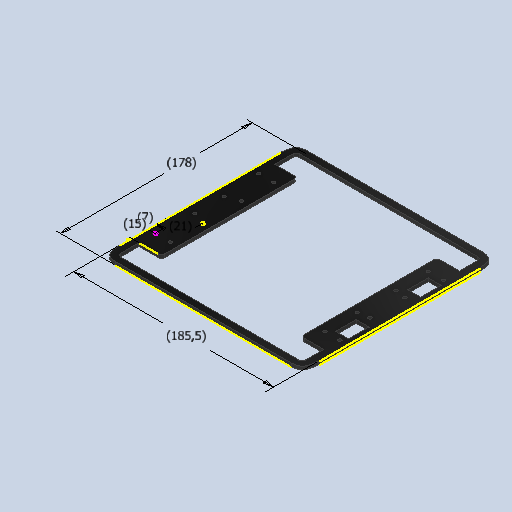
# Autodesk Inventor part: rama
Saved by Autodesk Inventor 2022 (Build 260153000, 153)
## iProperties
Created: 2022-07-21
Part Number: rama
Material: Серебро
Document SubType Name: Modeling
Designer: akapu
Density: 10.49 g/cm^3
Appearance: Серебро
Author: akapu
Autodesk Inventor part; units mm, degrees
ref_plane "YZ Plane" through (0, 0, 0) normal (1, 0, 0) x (0, 1, 0)
ref_plane "XZ Plane" through (0, 0, 0) normal (0, 1, 0) x (-1, 0, 0)
ref_plane "XY Plane" through (0, 0, 0) normal (0, 0, 1) x (1, 0, 0)
sketch "Эскиз1" plane through (0, 0, 0) normal (0, 1, 0) x (-1, 0, 0)
  line L0 (0, 0) -> (-92.765, 0)
  line L1 (-92.765, 0) -> (-92.765, -66)
  line L2 (-92.765, -66) -> (0, -66)
  line L3 (0, -66) -> (0, 0)
  line L4 (0, 0) -> (-43, 0)
  line L5 (-43, 0) -> (-43, 1)
  line L6 (-43, 1) -> (-6, 1)
  line L7 (-6, 1) -> (-6, 16)
  line L8 (-6, 16) -> (-80, 16)
  line L9 (-80, 16) -> (-80, 1)
  line L10 (-80, 1) -> (-43, 1)
  line L11 (0, 0) -> (0, 17)
  line L12 (0, 17) -> (-92.765, 17)
  line L13 (-92.765, 17) -> (-92.765, 0)
  line L14 (0, 17) -> (0, 23)
  line L15 (0, 23) -> (-92.765, 23)
  line L16 (-92.765, 23) -> (-92.765, 17)
  line L17 (-43, 16) -> (-43, 23)
  line L18 (0, 0) -> (-7, 0)
  line L19 (-7, 0) -> (-7, 17)
  line L20 (0, 0) -> (-8, 0)
  line L21 (-8, 0) -> (-8, -3)
  line L22 (-8, -3) -> (-92.765, -3)
  line L23 (-8, -3) -> (-8, -66)
  line L24 (-7, 17) -> (0, 23)
  line L25 (-3.5, 20) -> (-0.0714, 16)
  line L26 (-0.0714, 16) -> (-6.0714, 23)
  line L27 (0, 15.9167) -> (-3.5, 20)
  line L28 (-3.5, 20) -> (-6.0714, 23)
  spline S0 degree 3 poles (0, 8.5) (-1.6685, 20.9552) (-1.0245, 23.9091) (-21.5, 23) knots 0 0 0 0 1 1 1 1
  point P0 (-1.75, 17.9583)
  point P1 (-4.7857, 21.5)
  point P2 (-11.0558, 23)
  dimension "d68" = 43
  dimension "d71" = 1
  dimension "d72" = 37
  dimension "d74" = 74
  dimension "d75" = 17
  dimension "d76" = 6
  dimension "d77" = 7
  dimension "d78" = 8
  dimension "d79" = 3
  constraints: 58 end point, 15 point on line, 13 perpendicular, 6 midpoint, 3 parallel, 2 collinear, 2 horizontal, 4 other
  measures "d68" distance of L0.start L4.end
  measures "d71" distance of L4.end L5.end
  measures "d72" distance of L5.end L6.end
  measures "d74" distance of L7.end L8.end
  measures "d75" distance of L0.start L11.end
  measures "d76" distance of L11.end L14.end
  measures "d77" distance of L0.start L18.end
  measures "d78" distance of L0.start L20.end
  measures "d79" distance of L20.end L21.end
extrude "Выдавливание2" add sketch "Эскиз1" against normal blind 3 contours L3 L2 L23 L21 L0 | L0 L19 L6 L7 L8 L12 S0 L11 | L19 L8 L7 L6 | L12 L24 L25 S0 | L12 L17 L15 S0 L26 L24 | L25 L24 S0 | L12 L16 L15 L17 | L26 S0 L24
mirror "Зеркальное отражение1" about plane through (0, 0, -66) normal (0, 0, -1) of "Выдавливание2"
mirror "Зеркальное отражение2" about plane through (92.765, 0, -149) normal (1, 0, 0) of "Выдавливание2", "Зеркальное отражение1"
fillet "Сопряжение2" radius 3 4 edges at (7, -1.5, 17) (178.53, -1.5, 17) (178.53, -1.5, -149) (7, -1.5, -149)
sketch "Эскиз4" plane through (0, -3, 0) normal (0, -1, 0) x (1, 0, 0)
  line L0 (174.4742, -155) -> (11.0558, -155) projected
  line L1 (11.0558, 23) -> (174.4742, 23) projected
  line L2 (185.53, -140.5) -> (185.53, 8.5) projected
  line L3 (0, 8.5) -> (0, -140.5) projected
  point P0 (0, 0)
  dimension "d87" = 178
  measures "d87" distance between parallel lines of L0 L1
sketch "Эскиз5" plane through (0, 0, 0) normal (0, 1, 0) x (1, 0, 0)
  line L0 (8, 0) -> (8, 132) projected
  line L1 (8, 0) -> (8, 3)
  line L2 (8, 3) -> (177.53, 3)
  line L3 (177.53, 0) -> (177.53, 132) projected
  line L4 (8, 132.1275) -> (8, 129.1275)
  line L5 (8, 129.1275) -> (177.53, 129.1275)
  line L6 (8, 129.1275) -> (28, 129.1275)
  line L7 (28, 129.1275) -> (28, 3)
  line L8 (28, 3) -> (8, 3)
  line L9 (8, 3) -> (8, 129.1275)
  line L10 (177.53, 129.1275) -> (157.53, 129.1275)
  line L11 (157.53, 129.1275) -> (157.53, 3)
  line L12 (157.53, 3) -> (177.53, 3)
  line L13 (177.53, 3) -> (177.53, 129.1275)
  line L14 (28, 129.1275) -> (14, 129.1275)
  line L15 (14, 129.1275) -> (14, 3)
  line L16 (157.53, 129.1275) -> (171.53, 129.1275)
  line L17 (171.53, 129.1275) -> (171.53, 3)
  line L18 (164.53, 3) -> (164.53, 18)
  line L19 (164.53, 18) -> (178.53, 18)
  line L20 (164.53, 18) -> (164.53, 48)
  line L21 (164.53, 48) -> (178.53, 48)
  line L22 (185.53, 140.5) -> (185.53, -8.5) projected
  line L23 (178.53, 48) -> (178.53, 18)
  line L24 (164.53, 129.1275) -> (164.53, 114.1275)
  line L25 (164.53, 114.1275) -> (164.53, 84.1275)
  line L26 (164.53, 84.1275) -> (178.53, 84.1275)
  line L27 (178.53, 84.1275) -> (178.53, 114.1275)
  line L28 (178.53, 114.1275) -> (164.53, 114.1275)
  line L29 (21, 129.1275) -> (21, 114.1275)
  line L30 (21, 114.1275) -> (21, 84.1275)
  line L31 (21, 3) -> (21, 18)
  line L32 (21, 18) -> (21, 48)
  line L33 (21, 48) -> (7, 48)
  line L34 (21, 18) -> (7, 18)
  line L35 (7, 18) -> (7, 48)
  line L36 (21, 84.1275) -> (7, 84.1275)
  line L37 (7, 84.1275) -> (7, 114.1275)
  line L38 (7, 114.1275) -> (21, 114.1275)
  circle A0 centre (7, 114.1275) radius 1.5
  circle A1 centre (21, 114.1275) radius 1.5
  circle A2 centre (21, 84.1275) radius 1.5
  circle A3 centre (7, 18) radius 1.5
  circle A4 centre (21, 18) radius 1.5
  circle A5 centre (21, 48) radius 1.5
  circle A6 centre (164.53, 114.1275) radius 1.5
  circle A7 centre (178.53, 114.1275) radius 1.5
  circle A8 centre (178.53, 84.1275) radius 1.5
  circle A9 centre (164.53, 84.1275) radius 1.5
  circle A10 centre (164.53, 48) radius 1.5
  circle A11 centre (178.53, 48) radius 1.5
  circle A12 centre (178.53, 18) radius 1.5
  circle A13 centre (164.53, 18) radius 1.5
  arc A14 (10.584, 53.1837) -> (8.6151, 50.9779) centre (9.41, 52.25) ccw projected
  arc A15 (8.6151, 50.9779) -> (10.584, 53.1837) centre (9.41, 52.25) ccw projected
  arc A16 (10.584, 78.8163) -> (8.6151, 81.0221) centre (9.41, 79.75) ccw projected
  arc A17 (8.6151, 81.0221) -> (10.584, 78.8163) centre (9.41, 79.75) ccw projected
  arc A18 (8.6151, 81.0221) -> (10.584, 78.8163) centre (9.41, 79.75) ccw projected
  circle A19 centre (9.41, 52.25) radius 1.5
  circle A20 centre (9.41, 79.75) radius 1.5
  point P0 (0, 0)
  point P1 (177.53, 16.882)
  point P2 (177.53, 19.118)
  point P3 (177.53, 46.882)
  point P4 (177.53, 49.118)
  point P5 (177.53, 83.0095)
  point P6 (177.53, 85.2455)
  point P7 (177.53, 113.0095)
  point P8 (177.53, 115.2455)
  point P9 (8, 115.2455)
  point P10 (8, 113.0095)
  point P11 (8, 19.118)
  point P12 (8, 16.882)
  point P13 (8, 80.2618)
  point P14 (8, 79.2382)
  point P15 (8, 52.7618)
  point P16 (8, 51.7382)
  dimension "d90" = 3
  dimension "d91" = 3
  dimension "d92" = 20
  dimension "d93" = 20
  dimension "d94" = 14
  dimension "d95" = 14
  dimension "d96" = 15
  dimension "d97" = 14
  dimension "d98" = 30
  dimension "d99" = 15
  dimension "d100" = 30
  dimension "d101" = 15
  dimension "d102" = 30
  dimension "d103" = 15
  dimension "d104" = 30
  dimension "d105" = 14
  dimension "d106" = 14
  dimension "d107" = 14
  dimension "d108" = 3
  dimension "d109" = 3
  dimension "d110" = 3
  dimension "d112" = 3
  dimension "d113" = 3
  dimension "d114" = 3
  dimension "d116" = 3
  dimension "d117" = 3
  dimension "d118" = 3
  dimension "d119" = 3
  dimension "d120" = 3
  dimension "d121" = 3
  dimension "d122" = 3
  dimension "d123" = 3
  constraints: 72 end point, 17 point on line, 16 centre point, 16 coincident, 16 perpendicular, 6 parallel, 3 horizontal, 2 concentric, 2 midpoint, 1 vertical
  measures "d90" distance of L0.start L1.end
  measures "d91" distance of L4.start L4.end
  measures "d92" distance of L7.end L8.end
  measures "d93" distance of L12.end L11.end
  measures "d94" distance of L6.end L14.end
  measures "d95" distance of L10.end L16.end
  measures "d96" distance of L18.start L18.end
  measures "d97" distance of L18.end L19.end
  measures "d98" distance of L18.end L20.end
  measures "d99" distance of L24.start L24.end
  measures "d100" distance of L24.end L25.end
  measures "d101" distance of L29.start L29.end
  measures "d102" distance of L29.end L30.end
  measures "d103" distance of L31.start L31.end
  measures "d104" distance of L31.end L32.end
  measures "d105" distance of L32.end L33.end
  measures "d106" distance of L31.end L34.end
  measures "d107" distance of L30.end L36.end
  measures "d108" diameter of A0
  measures "d109" diameter of A1
  measures "d110" diameter of A2
  measures "d112" diameter of A3
  measures "d113" diameter of A4
  measures "d114" diameter of A5
  measures "d116" diameter of A6
  measures "d117" diameter of A7
  measures "d118" diameter of A8
  measures "d119" diameter of A9
  measures "d120" diameter of A10
  measures "d121" diameter of A11
  measures "d122" diameter of A12
  measures "d123" diameter of A13
extrude "Выдавливание3" add sketch "Эскиз5" against normal blind 3 contours L0 A3 L34 L15 L2 | L0 L34 A3 | L15 L34 A4 L31 L2 | L0 A3 L34 | A3 L0 L33 L15 L34 | L31 A4 L32 A5 L33 L15 L36 A2 L30 A1 L29 L5 L7 L2 | L15 L33 A5 L32 A4 L34 | L33 L0 A14 A15 A17 A16 L36 L15 | L11 L5 L24 A6 L25 A9 L26 L17 L21 A10 L20 A13 L18 L2 | L36 L0 A0 L38 L15 | L15 L38 A1 L30 A2 L36 | A14 L0 | L0 A14 A15 | L18 A13 L19 L17 L2 | L29 A1 L38 L15 L5 | L38 A0 L0 L5 L15 | L17 L19 A12 L3 L2 | L5 L17 L28 A6 L24 | A0 L0 L38 | L38 L0 A0 | A17 A16 L0 | L0 A17 | L19 A13 L20 A10 L21 L17 | L17 L21 A11 L3 A12 L19 | L5 L3 A7 L28 L17 | L17 L26 A8 L3 A11 L21 | L28 A7 L3 A8 L26 L17 | L17 L26 A9 L25 A6 L28
sketch "Эскиз6" plane through (0, 0, 0) normal (0, 1, 0) x (1, 0, 0)
  arc A0 (8, 16.882) -> (8, 19.118) centre (7, 18) ccw projected
  circle A1 centre (7, 18) radius 1.5
  arc A2 (8, 46.882) -> (8, 49.118) centre (7, 48) ccw projected
  circle A3 centre (7, 48) radius 1.5
  arc A4 (8, 83.0095) -> (8, 85.2455) centre (7, 84.1275) ccw projected
  circle A5 centre (7, 84.1275) radius 1.5
  arc A6 (8, 113.0095) -> (8, 115.2455) centre (7, 114.1275) ccw projected
  circle A7 centre (7, 114.1275) radius 1.5
  arc A8 (177.53, 115.2455) -> (177.53, 113.0095) centre (178.53, 114.1275) ccw projected
  circle A9 centre (178.53, 114.1275) radius 1.5
  arc A10 (177.53, 85.2455) -> (177.53, 83.0095) centre (178.53, 84.1275) ccw projected
  circle A11 centre (178.53, 84.1275) radius 1.5
  arc A12 (177.53, 49.118) -> (177.53, 46.882) centre (178.53, 48) ccw projected
  circle A13 centre (178.53, 48) radius 1.5
  arc A14 (177.53, 19.118) -> (177.53, 16.882) centre (178.53, 18) ccw projected
  circle A15 centre (178.53, 18) radius 1.5
  point P0 (0, 0)
  point P1 (177.53, 49.118)
  point P2 (177.53, 19.118)
  point P3 (8, 115.2455)
  point P4 (8, 85.2455)
  point P5 (8, 49.118)
  point P6 (8, 19.118)
  constraints: 8 coincident, 24 other
extrude "Выдавливание4" cut sketch "Эскиз6" against normal blind 3 contours A1 A0 | A7 A6 | A9 A8 | A11 A10 | A13 A12 | A15 A14
fillet "Сопряжение4" radius 3 4 edges at (28, -1.5, -3) (28, -1.5, -129.1275) (157.53, -1.5, -3) (157.53, -1.5, -129.1275)
sketch "Эскиз7" plane through (0, 0, 0) normal (0, 1, 0) x (1, 0, 0)
  line L0 (7, 0) -> (8, 0) projected
  line L1 (7, 0) -> (8, 0)
  line L2 (8, 0) -> (8, 3)
  line L3 (8, 3) -> (7, 3)
  line L4 (7, 3) -> (7, 0)
  line L5 (8, 129.1275) -> (8, 132) projected
  line L6 (7, 132) -> (8, 132) projected
  line L7 (8, 129.1275) -> (7, 129.1275)
  line L8 (7, 129.1275) -> (7, 132)
  line L9 (7, 132) -> (8, 132)
  line L10 (8, 132) -> (8, 129.1275)
  line L11 (178.53, 146) -> (178.53, 132) projected
  line L12 (177.53, 129.1275) -> (177.53, 132) projected
  line L13 (178.53, 132) -> (177.53, 132)
  line L14 (177.53, 132) -> (177.53, 129.1275)
  line L15 (177.53, 129.1275) -> (178.53, 129.1275)
  line L16 (178.53, 129.1275) -> (178.53, 132)
  line L17 (178.53, 0) -> (177.53, 0) projected
  line L18 (177.53, 0) -> (177.53, 3) projected
  line L19 (178.53, 0) -> (177.53, 0)
  line L20 (177.53, 0) -> (177.53, 3)
  line L21 (177.53, 3) -> (178.53, 3)
  line L22 (178.53, 3) -> (178.53, 0)
  point P0 (0, 0)
  constraints: 32 end point, 8 parallel, 4 horizontal, 4 perpendicular
extrude "Выдавливание5" cut sketch "Эскиз7" against normal blind 3
sketch "Эскиз8" plane through (0, 0, 0) normal (0, 1, 0) x (1, 0, 0)
  circle A0 centre (7, 18) radius 1.5 projected
  line L0 (7, 3) -> (25, 3) projected
  line L1 (0, 140.5) -> (0, -8.5) projected
  point P0 (0, 0)
  dimension "d131" = 15
  dimension "d132" = 7
  measures "d131" distance from line of A0.centre L0
  measures "d132" distance from line of A0.centre L1
sketch "Эскиз9" plane through (0, 0, 0) normal (0, 1, 0) x (1, 0, 0)
  line L0 (185.53, 140.5) -> (185.53, -8.5) projected
  line L1 (185.53, 66) -> (185.53, 96)
  line L2 (185.53, 96) -> (185.53, 36)
  line L3 (185.53, 36) -> (172.53, 36)
  line L4 (172.53, 36) -> (172.53, 96)
  line L5 (172.53, 96) -> (185.53, 96)
  point P0 (0, 0)
  dimension "d133" = 30
  dimension "d134" = 60
  dimension "d135" = 13
  constraints: 10 end point, 3 perpendicular, 2 point on line, 1 midpoint
  measures "d133" distance of L1.start L1.end
  measures "d134" distance of L1.end L2.end
  measures "d135" distance of L2.end L3.end
extrude "Выдавливание6" cut sketch "Эскиз9" against normal blind 3
fillet "Сопряжение5" radius 3 2 edges at (185.53, -1.5, -96) (185.53, -1.5, -36)
sketch "Эскиз11" plane through (0, 0, 0) normal (0, 1, 0) x (1, 0, 0)
  line L0 (185.53, 140.5) -> (185.53, 99) projected
  line L1 (0, -8.5) -> (0, 140.5) projected
  line L2 (185.53, 129.108) -> (0, 129.108)
  line L3 (0, 129.108) -> (0, 108.7964)
  line L4 (0, 108.7964) -> (185.53, 108.7964)
  line L5 (185.53, 108.7964) -> (185.53, 129.108)
  line L6 (172.53, 36) -> (172.53, 96) projected
  line L7 (0, 72.6312) -> (172.53, 72.6312)
  line L8 (172.53, 72.6312) -> (172.53, 96)
  line L9 (172.53, 96) -> (0, 96)
  line L10 (0, 96) -> (0, 72.6312)
  line L11 (185.53, 108.7964) -> (157.53, 108.7964)
  line L12 (157.53, 108.7964) -> (157.53, 129.108)
  line L13 (157.53, 129.108) -> (185.53, 129.108)
  line L14 (185.53, 129.108) -> (185.53, 108.7964)
  line L15 (157.53, 126.1275) -> (157.53, 6) projected
  line L16 (172.53, 72.6312) -> (157.53, 72.6312)
  line L17 (157.53, 72.6312) -> (157.53, 96)
  line L18 (157.53, 96) -> (172.53, 96)
  line L19 (172.53, 96) -> (172.53, 72.6312)
  line L20 (28, 6) -> (28, 126.1275) projected
  line L21 (0, 72.6312) -> (28, 72.6312)
  line L22 (28, 72.6312) -> (28, 96)
  line L23 (28, 96) -> (0, 96)
  line L24 (0, 96) -> (0, 72.6312)
  line L25 (28, 108.4447) -> (0, 108.4447)
  line L26 (0, 108.4447) -> (0, 129.108)
  line L27 (0, 129.108) -> (28, 129.108)
  line L28 (28, 129.108) -> (28, 108.4447)
  point P0 (0, 0)
  point P1 (0, 129.108)
  point P2 (28, 108.7964)
  point P3 (0, 96)
  constraints: 48 end point, 12 parallel, 9 point on line, 6 horizontal, 6 perpendicular
extrude "Выдавливание7" add sketch "Эскиз11" against normal blind 3 contours L0 L4 L12 L2 | L28 L20 L4 L1 L2 | L9 L6 L7 L15 | L20 L7 L1 L9
sketch "Эскиз10" plane through (0, 0, 0) normal (0, 1, 0) x (1, 0, 0)
  line L0 (25, 129.1275) -> (160.53, 129.1275) projected
  line L1 (160.53, 3) -> (178.53, 3) projected
  circle A0 centre (164.53, 114.1275) radius 1.5 projected
  circle A1 centre (164.53, 18) radius 1.5 projected
  circle A2 centre (164.53, 84.1275) radius 1.5 projected
  circle A3 centre (164.53, 48) radius 1.5 projected
  line L2 (172.53, 36) -> (172.53, 96) projected
  line L3 (172.53, 66) -> (164.53, 66)
  line L4 (164.53, 66) -> (164.53, 129)
  line L5 (164.53, 129) -> (178.53, 129)
  line L6 (178.53, 146) -> (178.53, 129.1275) projected
  line L7 (178.53, 129) -> (178.53, 129.1275)
  line L8 (7, 146) -> (7, 129.1275) projected
  line L9 (178.53, 129.1275) -> (7, 129.1275)
  line L10 (7, 129.1275) -> (7, 129)
  line L11 (7, 129) -> (164.53, 129)
  line L12 (164.53, 129) -> (164.53, 114)
  line L13 (164.53, 114) -> (164.53, 84)
  circle A4 centre (164.53, 84) radius 1.5
  circle A5 centre (164.53, 114) radius 1.5
  line L14 (7, 129) -> (7, 114)
  line L15 (7, 114) -> (7, 84)
  line L16 (7, 84) -> (21, 84)
  line L17 (21, 84) -> (21, 114)
  circle A6 centre (21, 114) radius 1.5
  circle A7 centre (7, 114) radius 1.5
  circle A8 centre (7, 84) radius 1.5
  circle A9 centre (21, 84) radius 1.5
  line L18 (164.53, 114) -> (178.53, 114)
  circle A10 centre (178.53, 114) radius 1.5
  point P0 (0, 0)
  dimension "d139" = 126.1275
  dimension "d140" = 96.1275
  dimension "d142" = 36.1275
  dimension "d143" = 63
  dimension "d144" = 15
  dimension "d145" = 30
  dimension "d146" = 3
  dimension "d147" = 3
  dimension "d148" = 15
  dimension "d149" = 30
  dimension "d150" = 3
  dimension "d151" = 3
  dimension "d152" = 3
  dimension "d153" = 3
  dimension "d158" = 3
  constraints: 28 end point, 8 perpendicular, 7 centre point, 7 coincident, 4 point on line, 2 horizontal, 1 midpoint, 1 vertical
  measures "d139" distance between parallel lines of L0 L1
  measures "d140" distance of A0.centre A1.centre
  measures "d142" distance of A2.centre A3.centre
  measures "d143" distance of L3.end L4.end
  measures "d144" distance of L4.end L12.end
  measures "d145" distance of L12.end L13.end
  measures "d146" diameter of A4
  measures "d147" diameter of A5
  measures "d148" distance of L10.end L14.end
  measures "d149" distance of L14.end L15.end
  measures "d150" diameter of A6
  measures "d151" diameter of A7
  measures "d152" diameter of A8
  measures "d153" diameter of A9
  measures "d158" diameter of A10
extrude "Выдавливание8" cut sketch "Эскиз10" against normal blind 3 contours L0 L9 L7 L5 L11 L10 | A5 L18 A0 | A0 L18 L4 A5 | A5 L4 A0 | A0 L4 A5 | L18 A5 L4 A0 | A0 L4 L18 | A4 L4 A2 | A2 L4 A4 | A4 L4 A2 | A2 L4 A4 | A7 L15 L14 | L14 L15 A7 | A9 L17 L16 | L16 L17 A9 | A6 | A10 picked at (164.2102, 114.9412) picked at (164.4158, 112.5557) picked at (164.6413, 82.555) picked at (165.046, 84.8496) picked at (164.2102, 84.9412) picked at (164.4158, 82.5557)
fillet "Сопряжение6" radius 3 2 edges at (28, -1.5, -129) (157.53, -1.5, -129)
sketch "Эскиз20" plane through (0, 0, 0) normal (0, 1, 0) x (1, 0, 0)
  arc A0 (182.53, 96) -> (185.53, 99) centre (182.53, 99) ccw projected
  line L0 (185.53, 99) -> (172.53, 99)
  line L1 (172.53, 99) -> (172.53, 32.217)
  line L2 (172.53, 32.217) -> (185.53, 32.217)
  line L3 (185.53, 32.217) -> (185.53, 99)
  point P0 (0, 0)
  constraints: 8 end point, 2 parallel, 1 horizontal, 1 perpendicular
extrude "Выдавливание12" add sketch "Эскиз20" against normal blind 3
sketch "Эскиз21" plane through (0, 0, 0) normal (0, 1, 0) x (1, 0, 0)
  line L0 (185.53, 140.5) -> (185.53, -8.5) projected
  line L1 (185.53, 66) -> (185.53, 82.227)
  line L2 (185.53, 66) -> (185.53, 49.773)
  line L3 (174.53, 49.773) -> (174.53, 82.227)
  line L4 (174.53, 49.773) -> (174.53, 42.022)
  line L5 (174.53, 42.022) -> (181.53, 42.022)
  line L6 (181.53, 42.022) -> (169.53, 42.022)
  line L7 (174.53, 82.227) -> (174.53, 89.978)
  line L8 (174.53, 89.978) -> (181.53, 89.978)
  line L9 (181.53, 89.978) -> (169.53, 89.978)
  circle A0 centre (178.53, 114) radius 1.5 projected
  line L10 (178.53, 108) -> (181.53, 108)
  line L11 (181.53, 108) -> (181.53, 89.978)
  line L12 (169.53, 89.978) -> (169.53, 108)
  line L13 (169.53, 108) -> (178.53, 108)
  circle A1 centre (178.53, 18) radius 1.5 projected
  line L14 (178.53, 24) -> (181.53, 24)
  line L15 (181.53, 24) -> (181.53, 42.022)
  line L16 (169.53, 42.022) -> (169.53, 24)
  line L17 (169.53, 24) -> (178.53, 24)
  line L18 (185.53, 66) -> (174.53, 66)
  line L19 (174.53, 66) -> (174.53, 82.23)
  line L20 (174.53, 82.23) -> (174.53, 49.77)
  circle A2 centre (174.53, 82.23) radius 1.6
  circle A3 centre (174.53, 49.77) radius 1.6
  point P0 (0, 0)
  dimension "d183" = 11
  dimension "d186" = 7.751
  dimension "d187" = 7
  dimension "d188" = 12
  dimension "d189" = 7.751
  dimension "d190" = 6
  dimension "d191" = 6
  dimension "d202" = 16.23
  dimension "d203" = 32.46
  dimension "d204" = 3.2
  dimension "d205" = 3.2
  constraints: 40 end point, 8 point on line, 6 perpendicular, 4 coincident, 2 centre point, 2 midpoint, 2 parallel, 1 vertical
  measures "d183" distance of L2.end L3.start
  measures "d186" distance of L4.start L4.end
  measures "d187" distance of L4.end L5.end
  measures "d188" distance of L5.end L6.end
  measures "d189" distance of L7.start L7.end
  measures "d190" distance of A0.centre L10.start
  measures "d191" distance of A1.centre L14.start
  measures "d202" distance of L18.end L19.end
  measures "d203" distance of L19.end L20.end
  measures "d204" diameter of A2
  measures "d205" diameter of A3
extrude "Выдавливание13" cut sketch "Эскиз21" against normal blind 3 contours L4 A3 L3 | L3 A3 L4 | A2 L7 L3 | L3 L7 A2 | L5 L15 L14 L17 L16 L6 | L9 L12 L13 L10 L11 L8
sketch "Эскиз22" plane through (0, 0, 0) normal (0, 1, 0) x (1, 0, 0)
  line L0 (181.53, 24) -> (169.53, 24) projected
  line L1 (169.53, 24) -> (181.53, 24)
  line L2 (181.53, 24) -> (181.53, 23)
  line L3 (181.53, 23) -> (169.53, 23)
  line L4 (169.53, 23) -> (169.53, 24)
  line L5 (169.53, 108) -> (181.53, 108) projected
  line L6 (169.53, 108) -> (181.53, 108)
  line L7 (181.53, 108) -> (181.53, 109)
  line L8 (181.53, 109) -> (169.53, 109)
  line L9 (169.53, 109) -> (169.53, 108)
  point P0 (0, 0)
  dimension "d194" = 1
  dimension "d195" = 1
  constraints: 16 end point, 4 parallel, 2 horizontal, 2 perpendicular, 1 point on line
  measures "d194" distance of L1.end L2.end
  measures "d195" distance of L7.end L6.end
extrude "Выдавливание14" cut sketch "Эскиз22" against normal blind 3
sketch "Эскиз26" plane through (0, -3, 0) normal (0, -1, 0) x (1, 0, 0)
  arc A0 (8.6151, -50.9779) -> (10.584, -53.1837) centre (9.41, -52.25) ccw projected
  arc A1 (10.584, -53.1837) -> (8.6151, -50.9779) centre (9.41, -52.25) ccw projected
  arc A2 (10.584, -78.8163) -> (8.6151, -81.0221) centre (9.41, -79.75) ccw projected
  arc A3 (8.6151, -81.0221) -> (10.584, -78.8163) centre (9.41, -79.75) ccw projected
  circle A4 centre (9.41, -52.25) radius 1.5
  circle A5 centre (9.41, -79.75) radius 1.5
  point P0 (0, 0)
  constraints: 2 centre point, 2 coincident, 2 concentric
extrude "Выдавливание15" cut sketch "Эскиз26" against normal blind 3
sketch "Эскиз27" plane through (0, 0, 0) normal (0, 1, 0) x (1, 0, 0)
  line L0 (0, -8.5) -> (0.03, -8.5)
  line L1 (0.03, -8.5) -> (0.03, -8.7882)
  line L2 (0.03, -8.7882) -> (0, -8.7882)
  line L3 (0, -8.7882) -> (0, 141.4509)
  line L4 (0, 141.4509) -> (0.03, 141.4509)
  line L5 (0.03, 141.4509) -> (0.03, -8.7882)
  point P0 (0, 0)
  dimension "d208" = 0.03
  constraints: 12 end point, 2 horizontal, 2 parallel, 1 perpendicular, 1 vertical
  measures "d208" distance of L0.start L0.end
extrude "Выдавливание16" cut sketch "Эскиз27" against normal blind 3
sketch "Эскиз24" plane through (0, 0, 0) normal (0, 1, 0) x (1, 0, 0)
  circle A0 centre (21, 48) radius 1.5 projected
  line L0 (0, 140.5) -> (0, -8.5) projected
  line L1 (185.53, 140.5) -> (185.53, -8.5) projected
  line L2 (0.03, 140.7248) -> (0.03, -8.7248) projected
  point P0 (0, 0)
  dimension "d199" = 21
  dimension "d211" = 185.5
  measures "d199" distance from line of A0.centre L0
  measures "d211" distance between parallel lines of L1 L2
